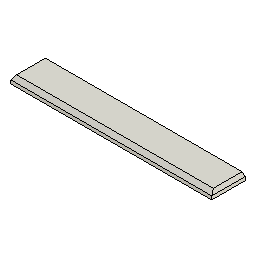
Choc v1 Spacebar v1 (Autodesk Fusion 360 design; units mm, degrees)
Autodesk Fusion 360 part; units mm, degrees
sketch "Base" plane through (0, 0, 0) normal (0, 0, 1) x (1, 0, 0)
  line L0 (49.5, -8.35) -> (-49.5, -8.35)
  line L1 (-49.5, -8.35) -> (-49.5, 8.35)
  line L2 (-49.5, 8.35) -> (49.5, 8.35)
  line L3 (49.5, 8.35) -> (49.5, -8.35)
  line L4 (49.5, -8.35) -> (-49.5, 8.35) construction
  line L5 (-49.5, -8.35) -> (49.5, 8.35) construction
  line L6 (13, 15) -> (14, 15)
  line L7 (49.3, 9.35) -> (-49.3, 9.35)
  line L8 (-50.5, 8.15) -> (-50.5, -8.15)
  line L9 (-49.3, -9.35) -> (49.3, -9.35)
  line L10 (50.5, -8.15) -> (50.5, 8.15)
  line L11 (50.5, 9.35) -> (-50.5, -9.35) construction
  line L12 (-50.5, 9.35) -> (50.5, -9.35) construction
  arc A0 (49.3, -9.35) -> (50.5, -8.15) centre (49.3, -8.15) ccw
  arc A1 (50.5, 8.15) -> (49.3, 9.35) centre (49.3, 8.15) ccw
  arc A2 (-49.3, 9.35) -> (-50.5, 8.15) centre (-49.3, 8.15) ccw
  arc A3 (-50.5, -8.15) -> (-49.3, -9.35) centre (-49.3, -8.15) ccw
  dimension "Depth" = 16.7
  dimension "Width" = 99
  dimension "OuterHoleGap" = 1
  dimension "d35" = 18.7
  dimension "d36" = 101
  dimension "d37" = 1.2
  constraint horizontal L0
  constraint perpendicular L0 L1
  constraint parallel L0 L2
  constraint parallel L1 L3
  constraint coincident L4 origin
  constraint coincident L5 origin
  constraint perpendicular L1 L6
  constraint horizontal L7
  constraint perpendicular L7 L8
  constraint parallel L7 L9
  constraint parallel L8 L10
  constraint coincident L11 origin
  constraint coincident L12 origin
  constraint coincident L12.end L9
  constraint coincident L12.end L10
  constraint tangent L9 A0
  constraint tangent L10 A0
  constraint coincident L11.start L10
  constraint coincident L11.start L7
  constraint tangent L10 A1
  constraint tangent L7 A1
  constraint equal A0 A1
  constraint coincident L12.start L7
  constraint coincident L12.start L8
  constraint tangent L7 A2
  constraint tangent L8 A2
  constraint equal A0 A2
  constraint coincident L11.end L8
  constraint coincident L11.end L9
  constraint tangent L8 A3
  constraint tangent L9 A3
  constraint equal A0 A3
  measures "Depth" distance of L0.start L2.end
  measures "Width" distance of L0.start L0.end
  measures "OuterHoleGap" distance of L6.start L6.end
  measures "d35" distance of L11.start L12.end
  measures "d36" distance of L11.start L12.start
  measures "d37" radius of A0
extrude "Extrude1" add sketch "Base" along normal blind 1.6 draft -5 contours L0 L1 L2 L3 makes body 1
extrude "Extrude2" add 1 faces at (16.4533, -2.7367, 1.6) along direction (0, 0, 1) blind 1.8 separate body on bodies 1 makes body 2
draft "Draft1" angle -45 neutral plane through (0, 0, 1.6) pull (0, 0, -1) 1 faces at (16.4533, -8.21, 2.8) on bodies 2
draft "Draft2" angle -15 neutral plane through (0, 0, 1.6) pull (0, 0, -1) 1 faces at (-16.4533, 8.21, 2.8) on bodies 2
draft "Draft3" angle -30 neutral plane through (0, 0, 1.6) pull (0, 0, -1) 2 faces at (-49.36, -2.1367, 2.2) (49.36, -2.1367, 2.2) on bodies 2
combine "Combine3" operation add target body 1 tool bodies 2
shell "Shell1" thickness 0.7 removed faces 1 at (16.5, -2.7833, 0) on bodies 1
copy_body "CopyPasteBodies2" bodies 1 makes body 3
extrude "Extrude4" add 1 faces at (-16.2658, 8.1158, 0) along direction (0, 0, -1) blind 3 on bodies 3 bodies 3
fillet "Fillet2" radius 0.5 8 edges at (-49.5, -8.35, -1.5) (-49.43, -8.28, 0.8) (-49.5, 8.35, -1.5) (-49.43, 8.28, 0.8) (49.5, 8.35, -1.5) (49.43, 8.28, 0.8) (49.5, -8.35, -1.5) (49.43, -8.28, 0.8) on bodies 3
extrude "Extrude5" add sketch "Base" along normal blind 10 and the other way blind 3.3 separate body contours L0 L1 L2 L3 | L7 L8 L9 L10 A0 A1 A2 A3 makes body 4
copy_body "CopyPasteBodies3" bodies 4 makes body 5
move_body "Move2" bodies 1 3 4 5 to x (1, 0, 0) y (0, 1, 0) z (0, 0, 1) at (0, 0, 0)
hidden bodies 3 4 5
equation "FilletR = 0.2 mm"
equation "Travel = 3 mm"
equation "Thickness = 0.7 mm"
equation "StrokeTolerance = 0.3 mm"
equation "d33 = FilletR + StrokeTolerance"
equation "d35 = Depth + OuterHoleGap * 2"
equation "d36 = Width + OuterHoleGap * 2"
equation "d37 = FilletR + OuterHoleGap"
equation "d40 = Travel + StrokeTolerance"
equation "LayoutAngle = 0.0 deg"
named bodies: "Placeholder", "MEV", "Hole", "Territory"
